Autodesk Inventor part; units mm, degrees
(part 3 of 4)
sketch "スケッチ23" plane through (0, 0, -5) normal (0, 0, -1) x (-1, 0, 0)
  arc A0 (-100.8254, -50.5622) -> (-98.047, -47.0317) centre (-111.885, -39) ccw projected
  arc A1 (-97.8265, -46.769) -> (-98.047, -47.0317) centre (-97.1821, -47.5337) ccw projected
  line L0 (-97.8265, -46.769) -> (-59.9457, -14.8489) projected
  arc A2 (-58.3014, -15.6137) -> (-59.9457, -14.8489) centre (-59.3014, -15.6137) ccw projected
  line L1 (-58.3014, -15.6137) -> (-58.3014, -51.2848) projected
  arc A3 (-59.3014, -52.2848) -> (-58.3014, -51.2848) centre (-59.3014, -51.2848) ccw projected
  line L2 (-59.3014, -52.2848) -> (-100.1342, -52.2848) projected
  arc A4 (-100.8254, -50.5622) -> (-100.1342, -52.2848) centre (-100.1342, -51.2848) ccw projected
  line L3 (-100.0095, -57.2848) -> (-59.3014, -57.2848) projected
  arc A5 (-58.3014, -58.2848) -> (-59.3014, -57.2848) centre (-59.3014, -58.2848) ccw projected
  line L4 (-58.3014, -58.2848) -> (-58.3014, -81.9487) projected
  arc A6 (-58.9251, -82.8752) -> (-58.3014, -81.9487) centre (-59.3014, -81.9487) ccw projected
  line L5 (-58.9251, -82.8752) -> (-63.9261, -84.9061) projected
  arc A7 (-65.1718, -84.4734) -> (-63.9261, -84.9061) centre (-64.3023, -83.9795) ccw projected
  arc A8 (-65.1718, -84.4734) -> (-72.5868, -76.7173) centre (-84.3014, -95.339) ccw projected
  line L6 (-72.5868, -76.7173) -> (-100.542, -59.1313) projected
  arc A9 (-100.0095, -57.2848) -> (-100.542, -59.1313) centre (-100.0095, -58.2848) ccw projected
  line L7 (-62.421, -88.6121) -> (-57.3632, -86.5581) projected
  arc A10 (-56.3726, -86.6955) -> (-57.3632, -86.5581) centre (-56.9869, -87.4846) ccw projected
  arc A11 (-56.3726, -86.6955) -> (-54.1956, -87.6694) centre (-53.3014, -82.75) ccw projected
  arc A12 (-53.3763, -88.5912) -> (-54.1956, -87.6694) centre (-54.3744, -88.6533) ccw projected
  arc A13 (-53.3763, -88.5912) -> (-53.1201, -89.9424) centre (-47.8869, -88.25) ccw projected
  arc A14 (-53.6916, -91.1751) -> (-53.1201, -89.9424) centre (-54.0715, -90.2501) ccw projected
  line L8 (-53.6916, -91.1751) -> (-54.9084, -91.675) projected
  arc A15 (-55.2884, -91.75) -> (-54.9084, -91.675) centre (-55.2884, -90.75) ccw projected
  line L9 (-55.2884, -91.75) -> (-61.7638, -91.75) projected
  arc A16 (-62.7437, -90.9495) -> (-61.7638, -91.75) centre (-61.7638, -90.75) ccw projected
  arc A17 (-62.7437, -90.9495) -> (-63.0125, -89.7908) centre (-84.3014, -95.339) ccw projected
  arc A18 (-62.421, -88.6121) -> (-63.0125, -89.7908) centre (-62.0448, -89.5386) ccw projected
  arc A19 (-94.6777, -12.8943) -> (-92.8272, -12.2945) centre (-95.8897, -6) ccw projected
  arc A20 (-91.9522, -12.2945) -> (-92.8272, -12.2945) centre (-92.3897, -13.1937) ccw projected
  arc A21 (-91.9522, -12.2945) -> (-83.3484, -10.2772) centre (-88.8897, -6) ccw projected
  arc A22 (-82.7234, -9.9022) -> (-83.3484, -10.2772) centre (-82.5568, -10.8882) ccw projected
  arc A23 (-82.7234, -9.9022) -> (-80.5008, -9.125) centre (-83.8897, -3) ccw projected
  arc A24 (-80.0167, -9) -> (-80.5008, -9.125) centre (-80.0167, -10) ccw projected
  line L10 (-80.0167, -9) -> (-74.3173, -9) projected
  arc A25 (-73.8332, -9.125) -> (-74.3173, -9) centre (-74.3173, -10) ccw projected
  arc A26 (-73.8332, -9.125) -> (-71.6106, -9.9022) centre (-70.4443, -3) ccw projected
  arc A27 (-70.9856, -10.2772) -> (-71.6106, -9.9022) centre (-71.7772, -10.8882) ccw projected
  arc A28 (-70.9856, -10.2772) -> (-68.4513, -12.3212) centre (-65.4443, -6) ccw projected
  arc A29 (-68.2365, -13.989) -> (-68.4513, -12.3212) centre (-68.8809, -13.2243) ccw projected
  line L11 (-68.2365, -13.989) -> (-83.5434, -26.8873) projected
  arc A30 (-84.9525, -26.7669) -> (-83.5434, -26.8873) centre (-84.1878, -26.1225) ccw projected
  line L12 (-84.9525, -26.7669) -> (-95.2693, -14.5236) projected
  arc A31 (-94.6777, -12.8943) -> (-95.2693, -14.5236) centre (-94.5046, -13.8792) ccw projected
  arc A32 (-97.1203, -16.9825) -> (-98.885, -17.6269) centre (-97.885, -17.6269) ccw projected
  line L13 (-97.1203, -16.9825) -> (-87.2466, -28.7001) projected
  arc A33 (-87.3669, -30.1091) -> (-87.2466, -28.7001) centre (-88.0113, -29.3444) ccw projected
  line L14 (-87.3669, -30.1091) -> (-94.615, -36.2167) projected
  arc A34 (-96.2374, -35.6607) -> (-94.615, -36.2167) centre (-95.2594, -35.452) ccw projected
  arc A35 (-96.2374, -35.6607) -> (-98.7086, -29.9236) centre (-111.885, -39) ccw projected
  arc A36 (-98.885, -29.3564) -> (-98.7086, -29.9236) centre (-97.885, -29.3564) ccw projected
  line L15 (-98.885, -29.3564) -> (-98.885, -17.6269) projected
  circle A37 centre (-47.8869, -88.25) radius 1.5 projected
  arc A38 (-46.177, -92.4125) -> (-47.885, -83.75) centre (-47.8869, -88.25) ccw projected
  line L16 (-47.885, -83.75) -> (-53.3014, -83.75) projected
  arc A39 (-54.3014, -82.75) -> (-53.3014, -83.75) centre (-53.3014, -82.75) ccw projected
  line L17 (-54.3014, -82.75) -> (-54.3014, -10.5578) projected
  arc A40 (-53.9457, -9.7931) -> (-54.3014, -10.5578) centre (-53.3014, -10.5578) ccw projected
  line L18 (-53.9457, -9.7931) -> (-49.4443, -6) projected
  line L19 (-49.4443, -6) -> (-49.4443, -3) projected
  line L20 (-49.4443, -3) -> (-52.4443, -3) projected
  arc A41 (-54.4443, -3) -> (-52.4443, -3) centre (-53.4443, -3) ccw projected
  line L21 (-54.4443, -3) -> (-57.4443, -3) projected
  line L22 (-57.4443, -3) -> (-57.4443, -6) projected
  arc A42 (-59.4443, -6) -> (-57.4443, -6) centre (-58.4443, -6) ccw projected
  line L23 (-59.4443, -6) -> (-64.4443, -6) projected
  arc A43 (-66.4443, -6) -> (-64.4443, -6) centre (-65.4443, -6) ccw projected
  line L24 (-66.4443, -6) -> (-66.4443, -3) projected
  line L25 (-66.4443, -3) -> (-69.4443, -3) projected
  arc A44 (-71.4443, -3) -> (-69.4443, -3) centre (-70.4443, -3) ccw projected
  line L26 (-71.4443, -3) -> (-82.8897, -3) projected
  arc A45 (-84.8897, -3) -> (-82.8897, -3) centre (-83.8897, -3) ccw projected
  line L27 (-84.8897, -3) -> (-87.8897, -3) projected
  line L28 (-87.8897, -3) -> (-87.8897, -6) projected
  arc A46 (-89.8897, -6) -> (-87.8897, -6) centre (-88.8897, -6) ccw projected
  line L29 (-89.8897, -6) -> (-94.8897, -6) projected
  arc A47 (-96.8897, -6) -> (-94.8897, -6) centre (-95.8897, -6) ccw projected
  line L30 (-96.8897, -6) -> (-96.8897, -3) projected
  line L31 (-96.8897, -3) -> (-99.8897, -3) projected
  arc A48 (-101.8897, -3) -> (-99.8897, -3) centre (-100.8897, -3) ccw projected
  line L32 (-101.8897, -3) -> (-104.885, -3) projected
  line L33 (-104.885, -3) -> (-104.885, -31.8586) projected
  arc A49 (-119.127, -45.896) -> (-104.885, -31.8586) centre (-111.885, -39) ccw projected
  line L34 (-119.127, -45.896) -> (-127.6513, -45.7727) projected
  line L35 (-127.6513, -45.7727) -> (-121.0577, -50.8686) projected
  arc A50 (-121.0577, -50.8686) -> (-119.8722, -51.6966) centre (-111.885, -39) ccw projected
  line L36 (-119.8722, -51.6966) -> (-74.7167, -80.1031) projected
  arc A51 (-66.3014, -95.339) -> (-74.7167, -80.1031) centre (-84.3014, -95.339) ccw projected
  line L37 (-66.3014, -95.339) -> (-66.3014, -95.75) projected
  line L38 (-66.3014, -95.75) -> (-54.3014, -95.75) projected
  line L39 (-54.3014, -95.75) -> (-46.177, -92.4125) projected
  line L40 (-98.885, -29.6726) -> (-98.885, -12.3268)
  arc A52 (-98.885, -12.3268) -> (-92.3897, -12.0622) centre (-95.8897, -6) ccw
  arc A53 (-92.3897, -12.0622) -> (-81.8897, -6) centre (-88.8897, -6) ccw
  line L41 (-81.8897, -6) -> (-81.8897, 3.7082)
  arc A54 (-81.8897, 3.7082) -> (-80.2841, -9) centre (-83.8897, -3) ccw
  line L42 (-80.2841, -9) -> (-74.0499, -9)
  arc A55 (-74.0499, -9) -> (-72.4443, 3.7082) centre (-70.4443, -3) ccw
  line L43 (-72.4443, 3.7082) -> (-72.4443, -6)
  arc A56 (-72.4443, -6) -> (-61.9443, 0.0622) centre (-65.4443, -6) ccw
  arc A57 (-61.9443, 0.0622) -> (-60.3014, -12.7492) centre (-58.4443, -6) ccw
  line L44 (-60.3014, -12.7492) -> (-60.3014, -82.75)
  arc A58 (-60.3014, -82.75) -> (-54.9853, -89.5444) centre (-53.3014, -82.75) ccw
  line L45 (-54.9853, -89.5444) -> (-55.4858, -89.75)
  line L46 (-55.4858, -89.75) -> (-60.9612, -89.75)
  arc A59 (-60.9612, -89.75) -> (-71.5218, -75.0244) centre (-84.3014, -95.339) ccw
  line L47 (-71.5218, -75.0244) -> (-116.6774, -46.618)
  arc A60 (-117.3886, -46.1211) -> (-116.6774, -46.618) centre (-111.885, -39) ccw
  line L48 (-117.3886, -46.1211) -> (-127.8557, -38.0317)
  arc A61 (-127.8557, -38.0317) -> (-98.885, -29.6726) centre (-111.885, -39) ccw
  line L49 (-94.615, -36.2167) -> (-87.3669, -30.1091) projected
  arc A62 (-84.9525, -26.7669) -> (-83.5434, -26.8873) centre (-84.1878, -26.1225) ccw projected
  line L50 (-87.3669, -30.1091) -> (-83.5434, -26.8873)
  point P0 (0, 0)
  point P1 (-94.6777, -12.8943)
  dimension "d189" = 6
  constraints: 20 end point, 20 point on circle, 10 centre point, 1 tangent, 18 other
  measures "d189" distance between parallel lines of L33 L40
extrude "押し出し25" cut sketch "スケッチ23" against normal blind 4 contours A33 L13 A32 L40 A52 A31 L12 A30 L50
fillet "フィレット7" radius 1 1 edges at (98.885, -12.3268, -3)
sketch "スケッチ24" plane through (0, 0, -5) normal (0, 0, -1) x (-1, 0, 0)
  arc A0 (-46.177, -92.4125) -> (-47.885, -83.75) centre (-47.8869, -88.25) ccw projected
  line L0 (-47.885, -83.75) -> (-53.3014, -83.75) projected
  arc A1 (-54.3014, -82.75) -> (-53.3014, -83.75) centre (-53.3014, -82.75) ccw projected
  line L1 (-54.3014, -82.75) -> (-54.3014, -10.5578) projected
  arc A2 (-53.9457, -9.7931) -> (-54.3014, -10.5578) centre (-53.3014, -10.5578) ccw projected
  line L2 (-53.9457, -9.7931) -> (-49.4443, -6) projected
  line L3 (-49.4443, -6) -> (-49.4443, -3) projected
  line L4 (-49.4443, -3) -> (-52.4443, -3) projected
  arc A3 (-54.4443, -3) -> (-52.4443, -3) centre (-53.4443, -3) ccw projected
  line L5 (-54.4443, -3) -> (-57.4443, -3) projected
  line L6 (-57.4443, -3) -> (-57.4443, -6) projected
  arc A4 (-59.4443, -6) -> (-57.4443, -6) centre (-58.4443, -6) ccw projected
  line L7 (-59.4443, -6) -> (-64.4443, -6) projected
  arc A5 (-66.4443, -6) -> (-64.4443, -6) centre (-65.4443, -6) ccw projected
  line L8 (-66.4443, -6) -> (-66.4443, -3) projected
  line L9 (-66.4443, -3) -> (-69.4443, -3) projected
  arc A6 (-71.4443, -3) -> (-69.4443, -3) centre (-70.4443, -3) ccw projected
  line L10 (-71.4443, -3) -> (-82.8897, -3) projected
  arc A7 (-84.8897, -3) -> (-82.8897, -3) centre (-83.8897, -3) ccw projected
  line L11 (-84.8897, -3) -> (-87.8897, -3) projected
  line L12 (-87.8897, -3) -> (-87.8897, -6) projected
  arc A8 (-89.8897, -6) -> (-87.8897, -6) centre (-88.8897, -6) ccw projected
  line L13 (-89.8897, -6) -> (-94.8897, -6) projected
  arc A9 (-96.8897, -6) -> (-94.8897, -6) centre (-95.8897, -6) ccw projected
  line L14 (-96.8897, -6) -> (-96.8897, -3) projected
  line L15 (-96.8897, -3) -> (-99.8897, -3) projected
  arc A10 (-101.8897, -3) -> (-99.8897, -3) centre (-100.8897, -3) ccw projected
  line L16 (-101.8897, -3) -> (-104.885, -3) projected
  line L17 (-104.885, -3) -> (-104.885, -31.8586) projected
  arc A11 (-119.127, -45.896) -> (-104.885, -31.8586) centre (-111.885, -39) ccw projected
  line L18 (-119.127, -45.896) -> (-127.6513, -45.7727) projected
  line L19 (-127.6513, -45.7727) -> (-121.0577, -50.8686) projected
  arc A12 (-121.0577, -50.8686) -> (-119.8722, -51.6966) centre (-111.885, -39) ccw projected
  line L20 (-119.8722, -51.6966) -> (-74.7167, -80.1031) projected
  arc A13 (-66.3014, -95.339) -> (-74.7167, -80.1031) centre (-84.3014, -95.339) ccw projected
  line L21 (-66.3014, -95.339) -> (-66.3014, -95.75) projected
  line L22 (-66.3014, -95.75) -> (-54.3014, -95.75) projected
  line L23 (-54.3014, -95.75) -> (-46.177, -92.4125) projected
  circle A14 centre (-47.8869, -88.25) radius 1.5 projected
  line L24 (-98.885, -29.3564) -> (-98.885, -13.7472) projected
  arc A15 (-97.6356, -12.7788) -> (-98.885, -13.7472) centre (-97.885, -13.7472) ccw projected
  arc A16 (-97.6356, -12.7788) -> (-92.8272, -12.2945) centre (-95.8897, -6) ccw projected
  arc A17 (-91.9522, -12.2945) -> (-92.8272, -12.2945) centre (-92.3897, -13.1937) ccw projected
  arc A18 (-91.9522, -12.2945) -> (-83.3484, -10.2772) centre (-88.8897, -6) ccw projected
  arc A19 (-82.7234, -9.9022) -> (-83.3484, -10.2772) centre (-82.5568, -10.8882) ccw projected
  arc A20 (-82.7234, -9.9022) -> (-80.5008, -9.125) centre (-83.8897, -3) ccw projected
  arc A21 (-80.0167, -9) -> (-80.5008, -9.125) centre (-80.0167, -10) ccw projected
  line L25 (-80.0167, -9) -> (-74.3173, -9) projected
  arc A22 (-73.8332, -9.125) -> (-74.3173, -9) centre (-74.3173, -10) ccw projected
  arc A23 (-73.8332, -9.125) -> (-71.6106, -9.9022) centre (-70.4443, -3) ccw projected
  arc A24 (-70.9856, -10.2772) -> (-71.6106, -9.9022) centre (-71.7772, -10.8882) ccw projected
  arc A25 (-70.9856, -10.2772) -> (-68.4513, -12.3212) centre (-65.4443, -6) ccw projected
  arc A26 (-68.2365, -13.989) -> (-68.4513, -12.3212) centre (-68.8809, -13.2243) ccw projected
  line L26 (-68.2365, -13.989) -> (-94.615, -36.2167) projected
  arc A27 (-96.2374, -35.6607) -> (-94.615, -36.2167) centre (-95.2594, -35.452) ccw projected
  arc A28 (-96.2374, -35.6607) -> (-98.7086, -29.9236) centre (-111.885, -39) ccw projected
  arc A29 (-98.885, -29.3564) -> (-98.7086, -29.9236) centre (-97.885, -29.3564) ccw projected
  line L27 (-62.421, -88.6121) -> (-57.3632, -86.5581) projected
  arc A30 (-56.3726, -86.6955) -> (-57.3632, -86.5581) centre (-56.9869, -87.4846) ccw projected
  arc A31 (-56.3726, -86.6955) -> (-54.1956, -87.6694) centre (-53.3014, -82.75) ccw projected
  arc A32 (-53.3763, -88.5912) -> (-54.1956, -87.6694) centre (-54.3744, -88.6533) ccw projected
  arc A33 (-53.3763, -88.5912) -> (-53.1201, -89.9424) centre (-47.8869, -88.25) ccw projected
  arc A34 (-53.6916, -91.1751) -> (-53.1201, -89.9424) centre (-54.0715, -90.2501) ccw projected
  line L28 (-53.6916, -91.1751) -> (-54.9084, -91.675) projected
  arc A35 (-55.2884, -91.75) -> (-54.9084, -91.675) centre (-55.2884, -90.75) ccw projected
  line L29 (-55.2884, -91.75) -> (-61.7638, -91.75) projected
  arc A36 (-62.7437, -90.9495) -> (-61.7638, -91.75) centre (-61.7638, -90.75) ccw projected
  arc A37 (-62.7437, -90.9495) -> (-63.0125, -89.7908) centre (-84.3014, -95.339) ccw projected
  arc A38 (-62.421, -88.6121) -> (-63.0125, -89.7908) centre (-62.0448, -89.5386) ccw projected
  line L30 (-100.0095, -57.2848) -> (-59.3014, -57.2848) projected
  arc A39 (-58.3014, -58.2848) -> (-59.3014, -57.2848) centre (-59.3014, -58.2848) ccw projected
  line L31 (-58.3014, -58.2848) -> (-58.3014, -81.9487) projected
  arc A40 (-58.9251, -82.8752) -> (-58.3014, -81.9487) centre (-59.3014, -81.9487) ccw projected
  line L32 (-58.9251, -82.8752) -> (-63.9261, -84.9061) projected
  arc A41 (-65.1718, -84.4734) -> (-63.9261, -84.9061) centre (-64.3023, -83.9795) ccw projected
  arc A42 (-65.1718, -84.4734) -> (-72.5868, -76.7173) centre (-84.3014, -95.339) ccw projected
  line L33 (-72.5868, -76.7173) -> (-100.542, -59.1313) projected
  arc A43 (-100.0095, -57.2848) -> (-100.542, -59.1313) centre (-100.0095, -58.2848) ccw projected
  arc A44 (-100.8254, -50.5622) -> (-98.047, -47.0317) centre (-111.885, -39) ccw projected
  arc A45 (-97.8265, -46.769) -> (-98.047, -47.0317) centre (-97.1821, -47.5337) ccw projected
  line L34 (-97.8265, -46.769) -> (-59.9457, -14.8489) projected
  arc A46 (-58.3014, -15.6137) -> (-59.9457, -14.8489) centre (-59.3014, -15.6137) ccw projected
  line L35 (-58.3014, -15.6137) -> (-58.3014, -51.2848) projected
  arc A47 (-59.3014, -52.2848) -> (-58.3014, -51.2848) centre (-59.3014, -51.2848) ccw projected
  line L36 (-59.3014, -52.2848) -> (-100.1342, -52.2848) projected
  arc A48 (-100.8254, -50.5622) -> (-100.1342, -52.2848) centre (-100.1342, -51.2848) ccw projected
  line L37 (-59.3014, -51.2848) -> (-97.885, -13.7472) construction
  line L38 (-58.2554, -50.2097) -> (-96.8391, -12.672)
  line L39 (-98.931, -14.8223) -> (-60.3473, -52.36)
  arc A49 (-60.3473, -52.36) -> (-58.2554, -50.2097) centre (-59.3014, -51.2848) ccw
  arc A50 (-96.8391, -12.672) -> (-98.931, -14.8223) centre (-97.885, -13.7472) ccw
  point P0 (0, 0)
  point P1 (-78.5932, -32.516)
  dimension "d193" = 3
  constraints: 8 end point, 4 point on circle, 4 tangent, 2 centre point, 1 midpoint, 1 parallel
  measures "d193" diameter of A50
extrude "押し出し26" add sketch "スケッチ24" against normal blind 5 contours L39 A50 L38 A16 A15 L24 | L24 A15 A16 L38 L26 L39 | L26 L38 L34 L39 | L34 L38 L35 A47 L36 L39 | L36 A47 L35 L38 A49 L39
fillet "フィレット8" radius 1 8 edges at (82.8384, -26.2932, -3) (85.1438, -28.2358, -3) (80.8221, -32.4403, -3) (78.5167, -30.4977, -3) (96.5323, -12.9704, -3) (98.885, -14.867, -3) (60.4246, -52.2848, -3) (58.3014, -50.1649, -3)
sketch "スケッチ25" plane through (0, 0, 0) normal (0, 0, 1) x (1, 0, 0)
  arc A0 (92.8272, -12.2945) -> (94.4295, -12.846) centre (95.8897, -6) ccw projected
  arc A1 (92.8272, -12.2945) -> (91.9522, -12.2945) centre (92.3897, -13.1937) ccw projected
  arc A2 (83.3484, -10.2772) -> (91.9522, -12.2945) centre (88.8897, -6) ccw projected
  arc A3 (83.3484, -10.2772) -> (82.7234, -9.9022) centre (82.5568, -10.8882) ccw projected
  arc A4 (80.5008, -9.125) -> (82.7234, -9.9022) centre (83.8897, -3) ccw projected
  arc A5 (80.5008, -9.125) -> (80.0167, -9) centre (80.0167, -10) ccw projected
  line L0 (80.0167, -9) -> (74.3173, -9) projected
  arc A6 (74.3173, -9) -> (73.8332, -9.125) centre (74.3173, -10) ccw projected
  arc A7 (71.6106, -9.9022) -> (73.8332, -9.125) centre (70.4443, -3) ccw projected
  arc A8 (71.6106, -9.9022) -> (70.9856, -10.2772) centre (71.7772, -10.8882) ccw projected
  arc A9 (68.4513, -12.3212) -> (70.9856, -10.2772) centre (65.4443, -6) ccw projected
  arc A10 (68.4513, -12.3212) -> (68.2365, -13.989) centre (68.8809, -13.2243) ccw projected
  line L1 (68.2365, -13.989) -> (82.1458, -25.7096) projected
  arc A11 (82.1458, -25.7096) -> (83.4875, -25.6616) centre (82.7902, -24.9449) ccw projected
  line L2 (83.4875, -25.6616) -> (94.9182, -14.5408) projected
  arc A12 (94.9182, -14.5408) -> (94.4295, -12.846) centre (94.2209, -13.824) ccw projected
  line L3 (77.6723, -29.7862) -> (59.9457, -14.8489) projected
  arc A13 (59.9457, -14.8489) -> (58.3014, -15.6137) centre (59.3014, -15.6137) ccw projected
  line L4 (58.3014, -15.6137) -> (58.3014, -47.7969) projected
  arc A14 (58.3014, -47.7969) -> (59.9987, -48.5136) centre (59.3014, -47.7969) ccw projected
  line L5 (59.9987, -48.5136) -> (77.7253, -31.2676) projected
  arc A15 (77.7253, -31.2676) -> (77.6723, -29.7862) centre (77.0279, -30.5509) ccw projected
  line L6 (97.1877, -16.5183) -> (85.9352, -27.4658) projected
  arc A16 (85.9352, -27.4658) -> (85.9881, -28.9473) centre (86.6325, -28.1826) ccw projected
  line L7 (85.9881, -28.9473) -> (94.615, -36.2167) projected
  arc A17 (94.615, -36.2167) -> (96.2374, -35.6607) centre (95.2594, -35.452) ccw projected
  arc A18 (98.7086, -29.9236) -> (96.2374, -35.6607) centre (111.885, -39) ccw projected
  arc A19 (98.7086, -29.9236) -> (98.885, -29.3564) centre (97.885, -29.3564) ccw projected
  line L8 (98.885, -29.3564) -> (98.885, -17.2351) projected
  arc A20 (98.885, -17.2351) -> (97.1877, -16.5183) centre (97.885, -17.2351) ccw projected
  line L9 (80.173, -33.0718) -> (62.1892, -50.5681) projected
  arc A21 (62.1892, -50.5681) -> (62.8865, -52.2848) centre (62.8865, -51.2848) ccw projected
  line L10 (62.8865, -52.2848) -> (100.1342, -52.2848) projected
  arc A22 (100.1342, -52.2848) -> (100.8254, -50.5622) centre (100.1342, -51.2848) ccw projected
  arc A23 (98.047, -47.0317) -> (100.8254, -50.5622) centre (111.885, -39) ccw projected
  arc A24 (98.047, -47.0317) -> (97.8265, -46.769) centre (97.1821, -47.5337) ccw projected
  line L11 (97.8265, -46.769) -> (81.5147, -33.0239) projected
  arc A25 (81.5147, -33.0239) -> (80.173, -33.0718) centre (80.8703, -33.7886) ccw projected
  arc A26 (47.885, -83.75) -> (46.177, -92.4125) centre (47.8869, -88.25) ccw projected
  line L12 (47.885, -83.75) -> (53.3014, -83.75) projected
  arc A27 (53.3014, -83.75) -> (54.3014, -82.75) centre (53.3014, -82.75) ccw projected
  line L13 (54.3014, -82.75) -> (54.3014, -10.5578) projected
  arc A28 (54.3014, -10.5578) -> (53.9457, -9.7931) centre (53.3014, -10.5578) ccw projected
  line L14 (53.9457, -9.7931) -> (49.4443, -6) projected
  line L15 (49.4443, -6) -> (49.4443, -3) projected
  line L16 (49.4443, -3) -> (52.4443, -3) projected
  arc A29 (52.4443, -3) -> (54.4443, -3) centre (53.4443, -3) ccw projected
  line L17 (54.4443, -3) -> (57.4443, -3) projected
  line L18 (57.4443, -3) -> (57.4443, -6) projected
  arc A30 (57.4443, -6) -> (59.4443, -6) centre (58.4443, -6) ccw projected
  line L19 (59.4443, -6) -> (64.4443, -6) projected
  arc A31 (64.4443, -6) -> (66.4443, -6) centre (65.4443, -6) ccw projected
  line L20 (66.4443, -6) -> (66.4443, -3) projected
  line L21 (66.4443, -3) -> (69.4443, -3) projected
  arc A32 (69.4443, -3) -> (71.4443, -3) centre (70.4443, -3) ccw projected
  line L22 (71.4443, -3) -> (82.8897, -3) projected
  arc A33 (82.8897, -3) -> (84.8897, -3) centre (83.8897, -3) ccw projected
  line L23 (84.8897, -3) -> (87.8897, -3) projected
  line L24 (87.8897, -3) -> (87.8897, -6) projected
  arc A34 (87.8897, -6) -> (89.8897, -6) centre (88.8897, -6) ccw projected
  line L25 (89.8897, -6) -> (94.8897, -6) projected
  arc A35 (94.8897, -6) -> (96.8897, -6) centre (95.8897, -6) ccw projected
  line L26 (96.8897, -6) -> (96.8897, -3) projected
  line L27 (96.8897, -3) -> (99.8897, -3) projected
  arc A36 (99.8897, -3) -> (101.8897, -3) centre (100.8897, -3) ccw projected
  line L28 (101.8897, -3) -> (104.885, -3) projected
  line L29 (104.885, -3) -> (104.885, -31.8586) projected
  arc A37 (104.885, -31.8586) -> (119.127, -45.896) centre (111.885, -39) ccw projected
  line L30 (119.127, -45.896) -> (127.6513, -45.7727) projected
  line L31 (127.6513, -45.7727) -> (121.0577, -50.8686) projected
  arc A38 (119.8722, -51.6966) -> (121.0577, -50.8686) centre (111.885, -39) ccw projected
  line L32 (119.8722, -51.6966) -> (74.7167, -80.1031) projected
  arc A39 (74.7167, -80.1031) -> (66.3014, -95.339) centre (84.3014, -95.339) ccw projected
  line L33 (66.3014, -95.339) -> (66.3014, -95.75) projected
  line L34 (66.3014, -95.75) -> (54.3014, -95.75) projected
  line L35 (54.3014, -95.75) -> (46.177, -92.4125) projected
  circle A40 centre (47.8869, -88.25) radius 1.5 projected
  line L36 (62.421, -88.6121) -> (57.3632, -86.5581) projected
  arc A41 (57.3632, -86.5581) -> (56.3726, -86.6955) centre (56.9869, -87.4846) ccw projected
  arc A42 (54.1956, -87.6694) -> (56.3726, -86.6955) centre (53.3014, -82.75) ccw projected
  arc A43 (54.1956, -87.6694) -> (53.3763, -88.5912) centre (54.3744, -88.6533) ccw projected
  arc A44 (53.1201, -89.9424) -> (53.3763, -88.5912) centre (47.8869, -88.25) ccw projected
  arc A45 (53.1201, -89.9424) -> (53.6916, -91.1751) centre (54.0715, -90.2501) ccw projected
  line L37 (53.6916, -91.1751) -> (54.9084, -91.675) projected
  arc A46 (54.9084, -91.675) -> (55.2884, -91.75) centre (55.2884, -90.75) ccw projected
  line L38 (55.2884, -91.75) -> (61.7638, -91.75) projected
  arc A47 (61.7638, -91.75) -> (62.7437, -90.9495) centre (61.7638, -90.75) ccw projected
  arc A48 (63.0125, -89.7908) -> (62.7437, -90.9495) centre (84.3014, -95.339) ccw projected
  arc A49 (63.0125, -89.7908) -> (62.421, -88.6121) centre (62.0448, -89.5386) ccw projected
  line L39 (58.3014, -58.2848) -> (58.3014, -81.9487) projected
  arc A50 (58.3014, -81.9487) -> (58.9251, -82.8752) centre (59.3014, -81.9487) ccw projected
  line L40 (58.9251, -82.8752) -> (63.9261, -84.9061) projected
  arc A51 (63.9261, -84.9061) -> (65.1718, -84.4734) centre (64.3023, -83.9795) ccw projected
  arc A52 (72.5868, -76.7173) -> (65.1718, -84.4734) centre (84.3014, -95.339) ccw projected
  line L41 (72.5868, -76.7173) -> (100.542, -59.1313) projected
  arc A53 (100.542, -59.1313) -> (100.0095, -57.2848) centre (100.0095, -58.2848) ccw projected
  line L42 (100.0095, -57.2848) -> (59.3014, -57.2848) projected
  arc A54 (59.3014, -57.2848) -> (58.3014, -58.2848) centre (59.3014, -58.2848) ccw projected
  point P0 (0, 0)
sketch "スケッチ26" plane through (0, 0, -5) normal (0, 0, -1) x (-1, 0, 0)
  line L0 (-104.885, -3) -> (-104.885, -31.8586) projected
  line L1 (-104.8897, -3) -> (-104.885, -3) projected
  line L2 (-124.1514, -30.3665) -> (-104.8897, -3) projected
  arc A0 (-124.1514, -30.3665) -> (-126.8081, -37.4821) centre (-111.885, -39) ccw projected
  line L3 (-127.6513, -45.7727) -> (-126.8081, -37.4821) projected
  line L4 (-119.127, -45.896) -> (-127.6513, -45.7727) projected
  arc A1 (-119.127, -45.896) -> (-104.885, -31.8586) centre (-111.885, -39) ccw projected
  circle A2 centre (-111.885, -39) radius 3 projected
  arc A3 (-121.6981, -32.0932) -> (-123.8235, -37.7857) centre (-111.885, -39) ccw
  line L5 (-121.6981, -32.0932) -> (-107.885, -12.468)
  line L6 (-107.885, -12.468) -> (-107.885, -33.2554)
  arc A4 (-117.6869, -42.9165) -> (-107.885, -33.2554) centre (-111.885, -39) ccw
  line L7 (-117.6869, -42.9165) -> (-124.3355, -42.8203)
  line L8 (-124.3355, -42.8203) -> (-123.8235, -37.7857)
  circle A5 centre (-111.885, -39) radius 8
  point P0 (0, 0)
  dimension "d197" = 3
  dimension "d198" = 5
  constraints: 8 end point, 4 point on circle, 3 centre point, 5 other
  measures "d197" distance between parallel lines of L3 L8
  measures "d198" radial gap between concentric circles of A2 A5
extrude "押し出し27" add sketch "スケッチ19" against normal blind 4 contours A30 L26 A29 L25 A28 L24 | A36 L29 A35 A34 A33 L28 A32 L27 A31 | A42 L33 A41 A40 A39 L32 A38 L31 A37 L30
sketch "スケッチ27" plane through (0, 0, 0) normal (0, 0, 1) x (1, 0, 0)
  arc A0 (92.8272, -12.2945) -> (94.4295, -12.846) centre (95.8897, -6) ccw projected
  arc A1 (92.8272, -12.2945) -> (91.9522, -12.2945) centre (92.3897, -13.1937) ccw projected
  arc A2 (83.3484, -10.2772) -> (91.9522, -12.2945) centre (88.8897, -6) ccw projected
  arc A3 (83.3484, -10.2772) -> (82.7234, -9.9022) centre (82.5568, -10.8882) ccw projected
  arc A4 (80.5008, -9.125) -> (82.7234, -9.9022) centre (83.8897, -3) ccw projected
  arc A5 (80.5008, -9.125) -> (80.0167, -9) centre (80.0167, -10) ccw projected
  line L0 (80.0167, -9) -> (74.3173, -9) projected
  arc A6 (74.3173, -9) -> (73.8332, -9.125) centre (74.3173, -10) ccw projected
  arc A7 (71.6106, -9.9022) -> (73.8332, -9.125) centre (70.4443, -3) ccw projected
  arc A8 (71.6106, -9.9022) -> (70.9856, -10.2772) centre (71.7772, -10.8882) ccw projected
  arc A9 (68.4513, -12.3212) -> (70.9856, -10.2772) centre (65.4443, -6) ccw projected
  arc A10 (68.4513, -12.3212) -> (68.2365, -13.989) centre (68.8809, -13.2243) ccw projected
  line L1 (68.2365, -13.989) -> (82.1458, -25.7096) projected
  arc A11 (82.1458, -25.7096) -> (83.4875, -25.6616) centre (82.7902, -24.9449) ccw projected
  line L2 (83.4875, -25.6616) -> (94.9182, -14.5408) projected
  arc A12 (94.9182, -14.5408) -> (94.4295, -12.846) centre (94.2209, -13.824) ccw projected
  line L3 (77.6723, -29.7862) -> (59.9457, -14.8489) projected
  arc A13 (59.9457, -14.8489) -> (58.3014, -15.6137) centre (59.3014, -15.6137) ccw projected
  line L4 (58.3014, -15.6137) -> (58.3014, -47.7969) projected
  arc A14 (58.3014, -47.7969) -> (59.9987, -48.5136) centre (59.3014, -47.7969) ccw projected
  line L5 (59.9987, -48.5136) -> (77.7253, -31.2676) projected
  arc A15 (77.7253, -31.2676) -> (77.6723, -29.7862) centre (77.0279, -30.5509) ccw projected
  line L6 (97.1877, -16.5183) -> (85.9352, -27.4658) projected
  arc A16 (85.9352, -27.4658) -> (85.9881, -28.9473) centre (86.6325, -28.1826) ccw projected
  line L7 (85.9881, -28.9473) -> (94.615, -36.2167) projected
  arc A17 (94.615, -36.2167) -> (96.2374, -35.6607) centre (95.2594, -35.452) ccw projected
  arc A18 (98.7086, -29.9236) -> (96.2374, -35.6607) centre (111.885, -39) ccw projected
  arc A19 (98.7086, -29.9236) -> (98.885, -29.3564) centre (97.885, -29.3564) ccw projected
  line L8 (98.885, -29.3564) -> (98.885, -17.2351) projected
  arc A20 (98.885, -17.2351) -> (97.1877, -16.5183) centre (97.885, -17.2351) ccw projected
  line L9 (80.173, -33.0718) -> (62.1892, -50.5681) projected
  arc A21 (62.1892, -50.5681) -> (62.8865, -52.2848) centre (62.8865, -51.2848) ccw projected
  line L10 (62.8865, -52.2848) -> (100.1342, -52.2848) projected
  arc A22 (100.1342, -52.2848) -> (100.8254, -50.5622) centre (100.1342, -51.2848) ccw projected
  arc A23 (98.047, -47.0317) -> (100.8254, -50.5622) centre (111.885, -39) ccw projected
  arc A24 (98.047, -47.0317) -> (97.8265, -46.769) centre (97.1821, -47.5337) ccw projected
  line L11 (97.8265, -46.769) -> (81.5147, -33.0239) projected
  arc A25 (81.5147, -33.0239) -> (80.173, -33.0718) centre (80.8703, -33.7886) ccw projected
  arc A26 (47.885, -83.75) -> (46.177, -92.4125) centre (47.8869, -88.25) ccw projected
  line L12 (47.885, -83.75) -> (53.3014, -83.75) projected
  arc A27 (53.3014, -83.75) -> (54.3014, -82.75) centre (53.3014, -82.75) ccw projected
  line L13 (54.3014, -82.75) -> (54.3014, -10.5578) projected
  arc A28 (54.3014, -10.5578) -> (53.9457, -9.7931) centre (53.3014, -10.5578) ccw projected
  line L14 (53.9457, -9.7931) -> (49.4443, -6) projected
  line L15 (49.4443, -6) -> (49.4443, -3) projected
  line L16 (49.4443, -3) -> (52.4443, -3) projected
  arc A29 (52.4443, -3) -> (54.4443, -3) centre (53.4443, -3) ccw projected
  line L17 (54.4443, -3) -> (57.4443, -3) projected
  line L18 (57.4443, -3) -> (57.4443, -6) projected
  arc A30 (57.4443, -6) -> (59.4443, -6) centre (58.4443, -6) ccw projected
  line L19 (59.4443, -6) -> (64.4443, -6) projected
  arc A31 (64.4443, -6) -> (66.4443, -6) centre (65.4443, -6) ccw projected
  line L20 (66.4443, -6) -> (66.4443, -3) projected
  line L21 (66.4443, -3) -> (69.4443, -3) projected
  arc A32 (69.4443, -3) -> (71.4443, -3) centre (70.4443, -3) ccw projected
  line L22 (71.4443, -3) -> (82.8897, -3) projected
  arc A33 (82.8897, -3) -> (84.8897, -3) centre (83.8897, -3) ccw projected
  line L23 (84.8897, -3) -> (87.8897, -3) projected
  line L24 (87.8897, -3) -> (87.8897, -6) projected
  arc A34 (87.8897, -6) -> (89.8897, -6) centre (88.8897, -6) ccw projected
  line L25 (89.8897, -6) -> (94.8897, -6) projected
  arc A35 (94.8897, -6) -> (96.8897, -6) centre (95.8897, -6) ccw projected
  line L26 (96.8897, -6) -> (96.8897, -3) projected
  line L27 (96.8897, -3) -> (99.8897, -3) projected
  arc A36 (99.8897, -3) -> (101.8897, -3) centre (100.8897, -3) ccw projected
  line L28 (101.8897, -3) -> (104.885, -3) projected
  line L29 (104.885, -3) -> (104.885, -31.8586) projected
  arc A37 (104.885, -31.8586) -> (119.127, -45.896) centre (111.885, -39) ccw projected
  line L30 (119.127, -45.896) -> (127.6513, -45.7727) projected
  line L31 (127.6513, -45.7727) -> (121.0577, -50.8686) projected
  arc A38 (119.8722, -51.6966) -> (121.0577, -50.8686) centre (111.885, -39) ccw projected
  line L32 (119.8722, -51.6966) -> (74.7167, -80.1031) projected
  arc A39 (74.7167, -80.1031) -> (66.3014, -95.339) centre (84.3014, -95.339) ccw projected
  line L33 (66.3014, -95.339) -> (66.3014, -95.75) projected
  line L34 (66.3014, -95.75) -> (54.3014, -95.75) projected
  line L35 (54.3014, -95.75) -> (46.177, -92.4125) projected
  circle A40 centre (47.8869, -88.25) radius 1.5 projected
  line L36 (62.421, -88.6121) -> (57.3632, -86.5581) projected
  arc A41 (57.3632, -86.5581) -> (56.3726, -86.6955) centre (56.9869, -87.4846) ccw projected
  arc A42 (54.1956, -87.6694) -> (56.3726, -86.6955) centre (53.3014, -82.75) ccw projected
  arc A43 (54.1956, -87.6694) -> (53.3763, -88.5912) centre (54.3744, -88.6533) ccw projected
  arc A44 (53.1201, -89.9424) -> (53.3763, -88.5912) centre (47.8869, -88.25) ccw projected
  arc A45 (53.1201, -89.9424) -> (53.6916, -91.1751) centre (54.0715, -90.2501) ccw projected
  line L37 (53.6916, -91.1751) -> (54.9084, -91.675) projected
  arc A46 (54.9084, -91.675) -> (55.2884, -91.75) centre (55.2884, -90.75) ccw projected
  line L38 (55.2884, -91.75) -> (61.7638, -91.75) projected
  arc A47 (61.7638, -91.75) -> (62.7437, -90.9495) centre (61.7638, -90.75) ccw projected
  arc A48 (63.0125, -89.7908) -> (62.7437, -90.9495) centre (84.3014, -95.339) ccw projected
  arc A49 (63.0125, -89.7908) -> (62.421, -88.6121) centre (62.0448, -89.5386) ccw projected
  line L39 (58.3014, -58.2848) -> (58.3014, -81.9487) projected
  arc A50 (58.3014, -81.9487) -> (58.9251, -82.8752) centre (59.3014, -81.9487) ccw projected
  line L40 (58.9251, -82.8752) -> (63.9261, -84.9061) projected
  arc A51 (63.9261, -84.9061) -> (65.1718, -84.4734) centre (64.3023, -83.9795) ccw projected
  arc A52 (72.5868, -76.7173) -> (65.1718, -84.4734) centre (84.3014, -95.339) ccw projected
  line L41 (72.5868, -76.7173) -> (100.542, -59.1313) projected
  arc A53 (100.542, -59.1313) -> (100.0095, -57.2848) centre (100.0095, -58.2848) ccw projected
  line L42 (100.0095, -57.2848) -> (59.3014, -57.2848) projected
  arc A54 (59.3014, -57.2848) -> (58.3014, -58.2848) centre (59.3014, -58.2848) ccw projected
  arc A55 (109.7028, -15.0506) -> (107.885, -15.6261) centre (108.885, -15.6261) ccw projected
  line L43 (107.885, -15.6261) -> (107.885, -23.7831) projected
  arc A56 (107.885, -23.7831) -> (109.4606, -24.6009) centre (108.885, -23.7831) ccw projected
  line L44 (109.4606, -24.6009) -> (113.2999, -21.8986) projected
  arc A57 (113.2999, -21.8986) -> (113.5421, -20.5053) centre (112.7243, -21.0809) ccw projected
  line L45 (113.5421, -20.5053) -> (109.7028, -15.0506) projected
  arc A58 (108.3095, -29.0797) -> (107.885, -29.8974) centre (108.885, -29.8974) ccw projected
  line L46 (107.885, -29.8974) -> (107.885, -30.5147) projected
  arc A59 (107.885, -30.5147) -> (109.2184, -31.4575) centre (108.885, -30.5147) ccw projected
  arc A60 (116.8906, -32.7594) -> (109.2184, -31.4575) centre (111.885, -39) ccw projected
  arc A61 (116.8906, -32.7594) -> (118.0918, -32.7971) centre (117.5163, -31.9794) ccw projected
  line L47 (118.0918, -32.7971) -> (120.017, -31.4421) projected
  arc A62 (120.017, -31.4421) -> (120.2592, -30.0488) centre (119.4414, -30.6244) ccw projected
  line L48 (120.2592, -30.0488) -> (116.4199, -24.5941) projected
  arc A63 (116.4199, -24.5941) -> (115.0266, -24.3519) centre (115.6022, -25.1696) ccw projected
  line L49 (115.0266, -24.3519) -> (108.3095, -29.0797) projected
  line L50 (120.4273, -42.8769) -> (123.2447, -42.8361) projected
  arc A64 (123.2447, -42.8361) -> (124.2252, -41.735) centre (123.2303, -41.8362) ccw projected
  line L51 (124.2252, -41.735) -> (123.8235, -37.7857) projected
  arc A65 (123.8235, -37.7857) -> (123.011, -34.5042) centre (111.885, -39) ccw projected
  arc A66 (123.011, -34.5042) -> (121.5083, -34.0611) centre (122.0839, -34.8788) ccw projected
  line L52 (121.5083, -34.0611) -> (119.8185, -35.2504) projected
  arc A67 (119.8185, -35.2504) -> (119.4487, -36.3939) centre (120.3941, -36.0681) ccw projected
  arc A68 (119.4653, -41.5573) -> (119.4487, -36.3939) centre (111.885, -39) ccw projected
  arc A69 (119.4653, -41.5573) -> (120.4273, -42.8769) centre (120.4128, -41.877) ccw projected
  line L53 (104.885, -3) -> (104.885, -31.8586) projected
  line L54 (104.8897, -3) -> (104.885, -3) projected
  line L55 (124.1514, -30.3665) -> (104.8897, -3) projected
  arc A70 (126.8081, -37.4821) -> (124.1514, -30.3665) centre (111.885, -39) ccw projected
  line L56 (127.6513, -45.7727) -> (126.8081, -37.4821) projected
  line L57 (119.127, -45.896) -> (127.6513, -45.7727) projected
  arc A71 (104.885, -31.8586) -> (119.127, -45.896) centre (111.885, -39) ccw projected
  circle A72 centre (111.885, -39) radius 3 projected
  point P0 (0, 0)
sketch "スケッチ28" plane through (0, 0, 0) normal (0, 0, 1) x (1, 0, 0)
  circle A0 centre (49.9722, -10.5) radius 3
  circle A1 centre (49.9722, -10.5) radius 4.5
  circle A2 centre (83.3769, -17.5) radius 13.85
  circle A3 centre (54.3769, -17.5) radius 13.85
  circle A4 centre (24.9722, -17.5) radius 13.85
  line L0 (34.3401, -6) -> (64.939, -6)
  circle A5 centre (90.0199, -69.8335) radius 3
  circle A6 centre (90.0199, -69.8335) radius 4.5
  point P0 (0, 0)
  dimension "d201" = 6
  dimension "d202" = 9
  dimension "d203" = 25
  dimension "d204" = 4.5
  dimension "d205" = 9
  constraints: 7 centre point, 2 coincident, 2 end point, 1 horizontal, 4 other
  measures "d201" diameter of A0
  measures "d202" diameter of A1
  measures "d203" horizontal distance of A0.centre A4.centre
  measures "d204" distance from line of L0 A0.centre
  measures "d205" diameter of A6
extrude "押し出し28" add sketch "スケッチ28" against normal blind 5 contours A0 | A1 | A5 | A6
hole "穴3" at (90.0199, -69.8335, 0) at (49.9722, -10.5, 0) direction (0, 0, -1) diameter 3 depth 12 tip angle 118
fillet "フィレット9" radius 1 7 edges at (94.0906, -67.9154, -2.5) (86.5284, -72.6726, -2.5) (85.7402, -68.4428, -3) (90.619, -65.3736, -3) (54.3014, -11.7283, -2.5) (49.4443, -6, -2.5) (49.4768, -6.0274, -2.5)
sketch "スケッチ29" plane through (0, 0, -5) normal (0, 0, -1) x (-1, 0, 0)
  line L0 (-98.044, -11.4998) -> (-82.0469, -27.0631)
  arc A0 (-82.0469, -27.0631) -> (-80.7052, -27.1111) centre (-81.3496, -26.3464) ccw
  line L1 (-80.7052, -27.1111) -> (-61.3064, -10.7647)
  arc A1 (-61.3064, -10.7647) -> (-61.9507, -9) centre (-61.9507, -10) ccw
  line L2 (-61.9507, -9) -> (-62.4443, -9)
  arc A2 (-62.4443, -9) -> (-63.0443, -9.2) centre (-62.4443, -10) ccw
  arc A3 (-69.1163, -7.5865) -> (-63.0443, -9.2) centre (-65.4443, -6) ccw
  arc A4 (-69.1163, -7.5865) -> (-70.1163, -6.9865) centre (-70.0342, -7.9832) ccw
  arc A5 (-72.8443, -6.2) -> (-70.1163, -6.9865) centre (-70.4443, -3) ccw
  arc A6 (-72.8443, -6.2) -> (-73.4443, -6) centre (-73.4443, -7) ccw
  line L3 (-73.4443, -6) -> (-80.8897, -6)
  arc A7 (-80.8897, -6) -> (-81.4897, -6.2) centre (-80.8897, -7) ccw
  arc A8 (-84.2178, -6.9865) -> (-81.4897, -6.2) centre (-83.8897, -3) ccw
  arc A9 (-84.2178, -6.9865) -> (-85.2178, -7.5865) centre (-84.2998, -7.9832) ccw
  arc A10 (-91.2897, -9.2) -> (-85.2178, -7.5865) centre (-88.8897, -6) ccw
  arc A11 (-91.2897, -9.2) -> (-91.8897, -9) centre (-91.8897, -10) ccw
  line L4 (-91.8897, -9) -> (-92.8897, -9)
  arc A12 (-92.8897, -9) -> (-93.4897, -9.2) centre (-92.8897, -10) ccw
  arc A13 (-97.0553, -9.8264) -> (-93.4897, -9.2) centre (-95.8897, -6) ccw
  arc A14 (-97.0553, -9.8264) -> (-98.044, -11.4998) centre (-97.3467, -10.783) ccw
  line L5 (-102.1316, -58.1313) -> (-90.9084, -65.1915)
  arc A15 (-90.9084, -65.1915) -> (-90.3112, -65.343) centre (-90.376, -64.3451) ccw
  arc A16 (-85.8458, -68.1521) -> (-90.3112, -65.343) centre (-90.0199, -69.8335) ccw
  arc A17 (-85.8458, -68.1521) -> (-85.4507, -68.6249) centre (-84.9182, -67.7784) ccw
  line L6 (-85.4507, -68.6249) -> (-72.5868, -76.7173)
  arc A18 (-65.1718, -84.4734) -> (-72.5868, -76.7173) centre (-84.3014, -95.339) ccw
  arc A19 (-65.1718, -84.4734) -> (-63.9261, -84.9061) centre (-64.3023, -83.9795) ccw
  line L7 (-63.9261, -84.9061) -> (-58.9251, -82.8752)
  arc A20 (-58.9251, -82.8752) -> (-58.3014, -81.9487) centre (-59.3014, -81.9487) ccw
  line L8 (-58.3014, -81.9487) -> (-58.3014, -57.2848)
  arc A21 (-58.3014, -57.2848) -> (-59.3014, -56.2848) centre (-59.3014, -57.2848) ccw
  line L9 (-59.3014, -56.2848) -> (-101.5991, -56.2848)
  arc A22 (-101.5991, -56.2848) -> (-102.1316, -58.1313) centre (-101.5991, -57.2848) ccw
  circle A23 centre (-90.0199, -69.8335) radius 1.5
  circle A24 centre (-49.9722, -10.5) radius 1.5
  line L10 (-54.3014, -14.878) -> (-54.3014, -82.75)
  arc A25 (-54.3014, -82.75) -> (-53.3014, -83.75) centre (-53.3014, -82.75) ccw
  line L11 (-53.3014, -83.75) -> (-47.8869, -83.75)
  arc A26 (-46.177, -92.4125) -> (-47.8869, -83.75) centre (-47.8869, -88.25) ccw
  line L12 (-46.177, -92.4125) -> (-54.3014, -95.75)
  line L13 (-54.3014, -95.75) -> (-66.3014, -95.75)
  line L14 (-66.3014, -95.75) -> (-66.3014, -95.339)
  arc A27 (-66.3014, -95.339) -> (-74.7167, -80.1031) centre (-84.3014, -95.339) ccw
  line L15 (-74.7167, -80.1031) -> (-85.8413, -73.1048)
  arc A28 (-85.8413, -73.1048) -> (-87.0367, -73.2026) centre (-86.3737, -73.9513) ccw
  arc A29 (-94.3483, -68.603) -> (-87.0367, -73.2026) centre (-90.0199, -69.8335) ccw
  arc A30 (-94.3483, -68.603) -> (-94.7777, -67.4831) centre (-95.3102, -68.3295) ccw
  line L16 (-94.7777, -67.4831) -> (-119.8722, -51.6966)
  arc A31 (-121.0577, -50.8686) -> (-119.8722, -51.6966) centre (-111.885, -39) ccw
  line L17 (-121.0577, -50.8686) -> (-127.6513, -45.7727)
  line L18 (-127.6513, -45.7727) -> (-119.127, -45.896)
  arc A32 (-119.127, -45.896) -> (-104.885, -31.8586) centre (-111.885, -39) ccw
  line L19 (-104.885, -31.8586) -> (-104.885, -3)
  line L20 (-104.885, -3) -> (-101.8897, -3)
  arc A33 (-101.8897, -3) -> (-99.8897, -3) centre (-100.8897, -3) ccw
  line L21 (-99.8897, -3) -> (-96.8897, -3)
  line L22 (-96.8897, -3) -> (-96.8897, -6)
  arc A34 (-96.8897, -6) -> (-94.8897, -6) centre (-95.8897, -6) ccw
  line L23 (-94.8897, -6) -> (-89.8897, -6)
  arc A35 (-89.8897, -6) -> (-87.8897, -6) centre (-88.8897, -6) ccw
  line L24 (-87.8897, -6) -> (-87.8897, -3)
  line L25 (-87.8897, -3) -> (-84.8897, -3)
  arc A36 (-84.8897, -3) -> (-82.8897, -3) centre (-83.8897, -3) ccw
  line L26 (-82.8897, -3) -> (-71.4443, -3)
  arc A37 (-71.4443, -3) -> (-69.4443, -3) centre (-70.4443, -3) ccw
  line L27 (-69.4443, -3) -> (-66.4443, -3)
  line L28 (-66.4443, -3) -> (-66.4443, -6)
  arc A38 (-66.4443, -6) -> (-64.4443, -6) centre (-65.4443, -6) ccw
  line L29 (-64.4443, -6) -> (-59.4443, -6)
  arc A39 (-59.4443, -6) -> (-57.4443, -6) centre (-58.4443, -6) ccw
  line L30 (-57.4443, -6) -> (-57.4443, -3)
  line L31 (-57.4443, -3) -> (-54.4443, -3)
  arc A40 (-54.4443, -3) -> (-52.4443, -3) centre (-53.4443, -3) ccw
  line L32 (-52.4443, -3) -> (-49.4443, -3)
  line L33 (-49.4443, -3) -> (-49.4443, -5.2165)
  arc A41 (-49.4443, -5.2165) -> (-48.7221, -6.1771) centre (-48.4443, -5.2165) ccw
  arc A42 (-52.6961, -14.082) -> (-48.7221, -6.1771) centre (-49.9722, -10.5) ccw
  arc A43 (-52.6961, -14.082) -> (-54.3014, -14.878) centre (-53.3014, -14.878) ccw
  line L34 (-81.5147, -33.0239) -> (-102.2194, -50.4706)
  arc A44 (-103.5253, -51.4545) -> (-102.2194, -50.4706) centre (-111.885, -39) ccw
  arc A45 (-103.5253, -51.4545) -> (-102.968, -53.2848) centre (-102.968, -52.2848) ccw
  line L35 (-102.968, -53.2848) -> (-61.8586, -53.2848)
  arc A46 (-61.8586, -53.2848) -> (-61.1613, -51.5681) centre (-61.8586, -52.2848) ccw
  line L36 (-61.1613, -51.5681) -> (-80.173, -33.0718)
  arc A47 (-80.173, -33.0718) -> (-81.5147, -33.0239) centre (-80.8703, -33.7886) ccw
  line L37 (-58.3014, -47.7969) -> (-58.3014, -15.6137)
  arc A48 (-58.3014, -15.6137) -> (-59.9457, -14.8489) centre (-59.3014, -15.6137) ccw
  line L38 (-59.9457, -14.8489) -> (-77.6723, -29.7862)
  arc A49 (-77.6723, -29.7862) -> (-77.7253, -31.2676) centre (-77.0279, -30.5509) ccw
  line L39 (-77.7253, -31.2676) -> (-59.9987, -48.5136)
  arc A50 (-59.9987, -48.5136) -> (-58.3014, -47.7969) centre (-59.3014, -47.7969) ccw
  line L40 (-84.4946, -28.8673) -> (-99.1877, -14.5726)
  arc A51 (-99.1877, -14.5726) -> (-100.885, -15.2893) centre (-99.885, -15.2893) ccw
  line L41 (-100.885, -15.2893) -> (-100.885, -31.7889)
  arc A52 (-100.885, -31.7889) -> (-100.7422, -32.304) centre (-99.885, -31.7889) ccw
  arc A53 (-98.9442, -40.2383) -> (-100.7422, -32.304) centre (-111.885, -39) ccw
  arc A54 (-98.9442, -40.2383) -> (-97.3043, -41.0982) centre (-97.9487, -40.3335) ccw
  line L42 (-97.3043, -41.0982) -> (-84.5476, -30.3488)
  arc A55 (-84.5476, -30.3488) -> (-84.4946, -28.8673) centre (-85.1919, -29.5841) ccw
  arc A56 (-62.7437, -90.9495) -> (-63.0125, -89.7908) centre (-84.3014, -95.339) ccw
  arc A57 (-62.7437, -90.9495) -> (-61.7638, -91.75) centre (-61.7638, -90.75) ccw
  line L43 (-61.7638, -91.75) -> (-55.2884, -91.75)
  arc A58 (-55.2884, -91.75) -> (-54.9084, -91.675) centre (-55.2884, -90.75) ccw
  line L44 (-54.9084, -91.675) -> (-53.6916, -91.1751)
  arc A59 (-53.6916, -91.1751) -> (-53.1201, -89.9424) centre (-54.0715, -90.2501) ccw
  arc A60 (-53.3763, -88.5912) -> (-53.1201, -89.9424) centre (-47.8869, -88.25) ccw
  arc A61 (-53.3763, -88.5912) -> (-54.1956, -87.6694) centre (-54.3744, -88.6533) ccw
  arc A62 (-56.3726, -86.6955) -> (-54.1956, -87.6694) centre (-53.3014, -82.75) ccw
  arc A63 (-56.3726, -86.6955) -> (-57.3632, -86.5581) centre (-56.9869, -87.4846) ccw
  line L45 (-57.3632, -86.5581) -> (-62.421, -88.6121)
  arc A64 (-62.421, -88.6121) -> (-63.0125, -89.7908) centre (-62.0448, -89.5386) ccw
  circle A65 centre (-47.8869, -88.25) radius 1.5
  point P0 (0, 0)
  point P1 (0, 0)
  constraints: 126 point on circle, 92 end point, 66 centre point, 17 horizontal, 11 vertical, 261 other
extrude "押し出し29" cut sketch "スケッチ29" against normal blind 4 contours A14 A13 A12 L4 A11 A10 A9 A8 A7 L3 A6 A5 A4 A3 A2 L2 A1 L1 A0 L0 | A22 L9 A21 L8 A20 L7 A19 A18 L6 A17 A16 A15 L5 | A47 L36 A46 L35 A45 A44 L34 | A55 L42 A54 A53 A52 L41 A51 L40